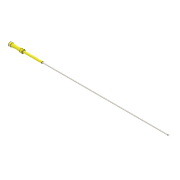
# Autodesk Inventor part: Nadel
Saved by Autodesk Inventor 2020.3 (Build 243373000, 373)
## iProperties
Created: 2022-01-03
Part Number: Nadel
Material: Generisch
Document SubType Name: Modeling
Designer: Sven
Density: 1 g/cm^3
Appearance: Vorgabe
Author: Sven
Autodesk Inventor part; units mm, degrees
ref_plane "YZ Plane" through (0, 0, 0) normal (1, 0, 0) x (0, 1, 0)
ref_plane "XZ Plane" through (0, 0, 0) normal (0, 1, 0) x (-1, 0, 0)
ref_plane "XY Plane" through (0, 0, 0) normal (0, 0, 1) x (1, 0, 0)
sketch "Skizze2" plane through (0, 0, 0) normal (0, 1, 0) x (-1, 0, 0)
  line L0 (0, 0) -> (0, -2.5)
  line L1 (0, -2.5) -> (3.2, -2.5)
  arc A0 (15.8, -2.5) -> (3.2, -2.5) centre (9.5, -24.1) ccw
  line L2 (15.8, -2.5) -> (19, -2.5)
  line L3 (19, -2.5) -> (19, 0)
  line L4 (19, 0) -> (0, 0)
  point P0 (9.5, -1.6)
  dimension "d5" = 2.5
  dimension "d6" = 2.5
  dimension "d7" = 3.2
  dimension "d8" = 3.2
  dimension "d9" = 19
  dimension "d10" = 0
  dimension "d11" = 1.6
  constraints: 10 end point, 3 point on circle, 2 perpendicular, 1 centre point, 1 horizontal, 1 vertical
  measures "d5" distance of L0.start L0.end
  measures "d6" distance from line of L3.end L2
  measures "d7" distance of L2.start L2.end
  measures "d8" distance of L0.end L1.end
  measures "d9" distance between parallel lines of L0 L3
  measures "d10" vertical distance of L0.start L3.end
  measures "d11" distance from line of L4 point (9.5, -1.6)
revolve "Umdrehung2" add sketch "Skizze2" angle 360 about axis through (-19, 0, 0) along (1, 0, 0)
sketch "Skizze3" plane through (-19, 0, 0) normal (-1, 0, 0) x (0, 0, 1)
  line L0 (5, -0.5) -> (-6, -0.5)
  line L1 (-6, -0.5) -> (-6, 0.5)
  line L2 (-6, 0.5) -> (5, 0.5)
  line L3 (5, 0.5) -> (5, -0.5)
  point P0 (0, 0)
  dimension "d13" = 0.5
  dimension "d14" = 0.5
  constraints: 8 end point, 2 parallel, 1 horizontal, 1 perpendicular
  measures "d13" distance from line of L0 point (0, 0)
  measures "d14" distance from line of point (0, 0) L2
extrude "Extrusion1" cut sketch "Skizze3" against normal blind 1.2
fillet "Rundung1" radius 0.5 4 edges at (-15.8, 0, 2.5) (-19, 2.5, 0) (-19, -2.5, 0) (0, 0, 2.5)
sketch "Skizze4" plane through (0, 0, 0) normal (1, 0, 0) x (0, 0, -1)
  circle A0 centre (0, 0) radius 1.25
  dimension "d18" = 2.5
  constraints: 1 centre point, 1 coincident
  measures "d18" diameter of A0
extrude "Extrusion2" add sketch "Skizze4" along normal blind 25.8
sketch "Skizze5" plane through (25.8, 0, 0) normal (1, 0, 0) x (0, 0, -1)
  circle A0 centre (0, 0) radius 2.4804 projected
  circle A1 centre (0, 0) radius 0.625
  dimension "d21" = 1.25
  constraints: 1 centre point, 1 coincident
  measures "d21" diameter of A1
extrude "Extrusion3" add sketch "Skizze5" along normal blind 176 contours A1
chamfer "Fase1" distance 0.6 distance2 3 1 edges at (201.8, 0, 0.625) measured on face at (201.8, -0.1535, -0.4143)
equation "\"d6\" = d5"
equation "\"d14\" = d13"
